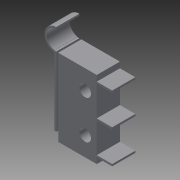
# Autodesk Inventor part: bumper
Saved by Autodesk Inventor 2015 (Build 190159000, 159)
## iProperties
Created: 2015-10-17
Part Number: bumper
Material: Générique
Document SubType Name: Modeling
Designer: astralien3000
Density: 1 g/cm^3
Appearance: Par défaut
Author: astralien3000
Autodesk Inventor part; units mm, degrees
ref_plane "YZ Plane" through (0, 0, 0) normal (1, 0, 0) x (0, 1, 0)
ref_plane "XZ Plane" through (0, 0, 0) normal (0, 1, 0) x (-1, 0, 0)
ref_plane "XY Plane" through (0, 0, 0) normal (0, 0, 1) x (1, 0, 0)
sketch "Esquisse1" plane through (0, 0, 0) normal (0, 1, 0) x (-1, 0, 0)
  line L0 (5, 10) -> (-5, 10)
  line L1 (-5, 10) -> (-5, -10)
  line L2 (-5, -10) -> (5, -10)
  line L3 (5, -10) -> (5, 10)
  point P0 (0, 0)
  dimension "d0" = 10
  dimension "d1" = 20
  dimension "d2" = 10
  dimension "d3" = 5
  constraints: 8 end point, 2 parallel, 1 horizontal, 1 perpendicular
  measures "d0" distance of L0.start L0.end
  measures "d1" distance of L2.end L0.start
  measures "d2" distance from line of L0 point (0, 0)
  measures "d3" distance from line of point (0, 0) L3
extrude "Extrusion1" add sketch "Esquisse1" along normal blind 6
sketch "Esquisse2" plane through (0, 6, 0) normal (0, 1, 0) x (1, 0, 0)
  circle A0 centre (2, -5) radius 1.5
  circle A1 centre (2, 5) radius 1.5
  line L0 (5, -10) -> (5, 10) projected
  line L1 (-5, -10) -> (5, -10) projected
  line L2 (5, 10) -> (-5, 10) projected
  point P0 (0, 0)
  dimension "d6" = 3
  dimension "d7" = 3
  dimension "d8" = 5
  dimension "d9" = 5
  dimension "d10" = 3
  dimension "d11" = 3
  constraints: 2 centre point
  measures "d6" distance from line of L0 A0.centre
  measures "d7" distance from line of L0 A1.centre
  measures "d8" distance from line of L1 A0.centre
  measures "d9" distance from line of L2 A1.centre
  measures "d10" diameter of A0
  measures "d11" diameter of A1
extrude "Extrusion2" cut sketch "Esquisse2" against normal through all
sketch "Esquisse3" plane through (5, 0, 10) normal (1, 0, 0) x (0, 0, -1)
  line L0 (1.5, 6) -> (2, 6)
  line L1 (2, 6) -> (2, 0)
  line L2 (2, 0) -> (1.5, 0)
  line L3 (1.5, 0) -> (1.5, 6)
  line L4 (18, 6) -> (18.5, 6)
  line L5 (18.5, 6) -> (18.5, 0)
  line L6 (18.5, 0) -> (18, 0)
  line L7 (18, 0) -> (18, 6)
  line L8 (9.75, 6) -> (10.25, 6)
  line L9 (10.25, 6) -> (10.25, 0)
  line L10 (10.25, 0) -> (9.75, 0)
  line L11 (9.75, 0) -> (9.75, 6)
  line L12 (0, 6) -> (20, 6) projected
  line L13 (0, 0) -> (20, 0) projected
  line L14 (0, 0) -> (0, 6) projected
  line L15 (20, 0) -> (20, 6) projected
  point P0 (10, 0)
  dimension "d14" = 1.5
  dimension "d15" = 1.5
  dimension "d16" = 0.5
  dimension "d17" = 0.5
  dimension "d18" = 0.5
  dimension "d19" = 16
  dimension "d20" = 7.75
  constraints: 24 end point, 6 parallel, 3 collinear, 3 horizontal, 3 perpendicular, 3 point on line
  measures "d14" distance between parallel lines of L14 L3
  measures "d15" distance between parallel lines of L15 L5
  measures "d16" distance between parallel lines of L7 L5
  measures "d17" distance between parallel lines of L3 L1
  measures "d18" distance between parallel lines of L9 L11
  measures "d19" distance between parallel lines of L7 L1
  measures "d20" distance between parallel lines of L7 L9
extrude "Extrusion3" add sketch "Esquisse3" along normal blind 4 contours L0 L1 L2 L3 | L8 L9 L10 L11 | L4 L5 L6 L7
sketch "Esquisse4" plane through (0, 6, 0) normal (0, 1, 0) x (1, 0, 0)
  line L0 (-6, 8) -> (-5.5, 8)
  line L1 (-5.5, 8) -> (-5.5, -9.5)
  line L2 (-5.5, -10) -> (-6, -10)
  line L3 (-6, -10) -> (-6, -9.542)
  line L4 (-5.5, -10) -> (-5.5, -15.5)
  arc A0 (-6, -10.0505) -> (-5.5, -15) centre (-5.5, -12.5) ccw
  arc A1 (-6, -9.542) -> (-5.5, -15.5) centre (-5.5, -12.5) ccw
  line L5 (-5, 10) -> (-5, -10) projected
  line L6 (5, 8) -> (9, 8) projected
  line L7 (-5, -10) -> (5, -10) projected
  line L8 (-6, -10) -> (-6, -10.0505)
  line L9 (-5.5, -9.5) -> (-5.5, -10)
  line L10 (-6, -9.542) -> (-6, 8)
  line L11 (-6, -10.0505) -> (-6, -15.458)
  arc A2 (-5.5, -10) -> (-6, -10.0505) centre (-5.5, -12.5) ccw
  arc A3 (-5.5, -9.5) -> (-6, -9.542) centre (-5.5, -12.5) ccw
  arc A4 (-5.5, -15) -> (-5.5, -10) centre (-5.5, -12.5) ccw
  arc A5 (-5.5, -15.5) -> (-5.5, -9.5) centre (-5.5, -12.5) ccw
  point P0 (0, 0)
  dimension "d23" = 0.5
  dimension "d24" = 0.5
  dimension "d25" = 0.5
  dimension "d27" = 5
  constraints: 18 end point, 14 point on circle, 6 centre point, 5 parallel, 3 vertical, 2 collinear, 2 perpendicular, 2 point on line, 1 coincident, 1 horizontal
  measures "d23" distance between parallel lines of L3 L1
  measures "d24" radial gap between concentric circles of A1 A0
  measures "d25" distance between parallel lines of L5 L1
  measures "d27" diameter of A0
extrude "Extrusion4" add sketch "Esquisse4" against normal blind 6 contours L0 L1 A3 L10 | A3 L9 L2 L3 | L3 L8 A0 L11 A1 | L11 A0 L4 A1
equation "\"d2\" = 0.5 * d1"
equation "\"d3\" = 0.5 * d0"
equation "\"d20\" = -0.5 * d18 + 0.5 * d19"
